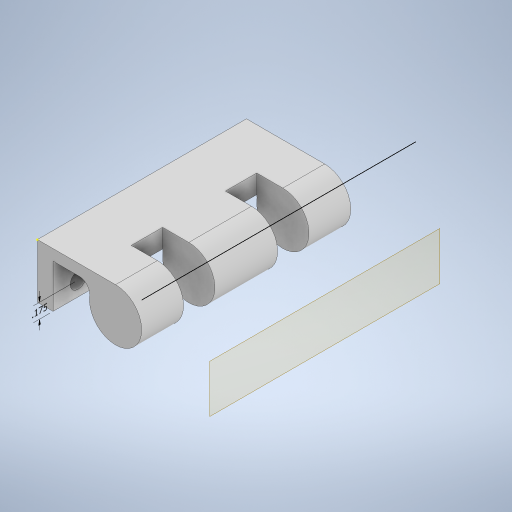
# Autodesk Inventor part: knuckle plate hinge tall
Saved by Autodesk Inventor 2024.2 (Build 282272000, 272)
## iProperties
Created: 2024-08-26
Part Number: knuckle plate hinge tall
Material: Generic
Document SubType Name: Modeling
Designer: Tom
Density: 1 g/cm^3
Appearance: Default
Author: Tom
Autodesk Inventor part; units mm, degrees
ref_plane "YZ Plane" through (0, 0, 0) normal (1, 0, 0) x (0, 1, 0)
ref_plane "XZ Plane" through (0, 0, 0) normal (0, 1, 0) x (-1, 0, 0)
ref_plane "XY Plane" through (0, 0, 0) normal (0, 0, 1) x (1, 0, 0)
sketch "Sketch1" plane through (0, 0, 0) normal (1, 0, 0) x (0, 1, 0)
  line L0 (0, 0) -> (16.51, 0)
  line L1 (16.51, 0) -> (16.51, -63.5)
  line L2 (16.51, -63.5) -> (0, -63.5)
  line L3 (0, -63.5) -> (0, 0)
  circle A0 centre (4.445, -7.62) radius 2.4329
  circle A1 centre (4.445, -15.6185) radius 2.4329
  circle A2 centre (4.445, -23.6169) radius 2.4329
  circle A3 centre (4.445, -31.6154) radius 2.4329
  circle A4 centre (4.445, -39.6138) radius 2.4329
  circle A5 centre (4.445, -47.6123) radius 2.4329
  circle A6 centre (4.445, -55.6108) radius 2.4329
  dimension "d0" = 63.5
  dimension "d1" = 16.51
  dimension "d6" = 7.9985
  dimension "d11" = 7.62
  constraints: 8 end point, 7 centre point, 2 parallel, 1 horizontal, 1 perpendicular, 1 vertical, 12 other
  measures "d0" distance of L0.end L1.end
  measures "d1" distance of L0.start L0.end
  measures "d6" distance of A0.centre A1.centre
  measures "d11" distance from line of L0 A0.centre
extrude "Extrusion1" add sketch "Sketch1" along normal blind 4.7625
sketch "Sketch2" plane through (4.7625, 0, 0) normal (1, 0, 0) x (0, 0, -1)
  line L0 (63.5, 16.51) -> (0, 16.51) projected
  line L1 (63.5, 0) -> (63.5, 16.51) projected
  line L2 (0, 16.51) -> (63.5, 16.51)
  line L3 (63.5, 16.51) -> (63.5, 13.208)
  line L4 (63.5, 13.208) -> (0, 13.208)
  line L5 (0, 13.208) -> (0, 16.51)
  point P0 (0, 0)
  dimension "d14" = 3.302
  constraints: 8 end point, 2 parallel, 1 horizontal, 1 perpendicular, 1 point on line
  measures "d14" distance between parallel lines of L4 L0
extrude "Extrusion2" add sketch "Sketch2" along normal blind 1.016
sketch "Sketch3" plane through (0, 0, 0) normal (0, 0, 1) x (1, 0, 0)
  line L0 (5.7785, 16.51) -> (5.7785, 13.208) projected
  arc A0 (15.8804, 9.6157) -> (23.749, 16.51) centre (23.749, 8.5725) ccw
  line L1 (0, 16.51) -> (0, 0) projected
  line L2 (5.7785, 16.51) -> (23.749, 16.51)
  line L3 (4.7625, 13.208) -> (5.7785, 13.208) projected
  line L4 (5.7785, 13.208) -> (12.7329, 13.208)
  arc A1 (15.8804, 9.6157) -> (12.7329, 13.208) centre (12.7329, 10.033) ccw
  point P0 (17.3057, 13.208)
  point P1 (9.5258, 13.208)
  dimension "d17" = 23.749
  dimension "d18" = 15.875
  dimension "d19" = 3.175
  constraints: 5 point on circle, 4 end point, 3 tangent, 2 centre point, 1 collinear, 1 horizontal, 1 point on line
  measures "d17" distance from line of L1 A0.centre
  measures "d18" diameter of A0
  measures "d19" radius of A1
extrude "Extrusion3" add sketch "Sketch3" against normal blind 63.5
sketch "Sketch4" plane through (0, 16.51, 0) normal (0, 1, 0) x (1, 0, 0)
  line L0 (31.6865, 0) -> (31.6865, 63.5) projected
  line L1 (31.6865, 0) -> (31.6865, 83.2403)
  point P0 (0, 0)
  constraints: 2 end point, 1 point on line, 1 vertical
ref_plane "Work Plane1" through (55.5625, 0, 0) normal (1, 0, 0) x (0, 0, -1)
sketch "Sketch6" plane through (0, 16.51, 0) normal (0, 1, 0) x (1, 0, 0)
  line L0 (31.6865, 0) -> (31.6865, 63.5) projected
  line L1 (15.8115, 50.8) -> (31.6865, 50.8)
  line L2 (31.6865, 50.8) -> (31.6865, 41.275)
  line L3 (31.6865, 41.275) -> (15.8115, 41.275)
  line L4 (15.8115, 41.275) -> (15.8115, 50.8)
  line L5 (31.6865, 63.5) -> (15.8115, 63.5) projected
  line L6 (15.8115, 22.225) -> (31.6865, 22.225)
  line L7 (31.6865, 22.225) -> (31.6865, 12.7)
  line L8 (31.6865, 12.7) -> (15.8115, 12.7)
  line L9 (15.8115, 12.7) -> (15.8115, 22.225)
  line L10 (15.8115, 0) -> (31.6865, 0) projected
  point P0 (0, 0)
  point P1 (15.8804, 63.5)
  point P2 (15.8804, 0)
  dimension "d26" = 9.525
  dimension "d27" = 12.7
  dimension "d28" = 9.525
  dimension "d29" = 12.7
  dimension "d32" = 15.875
  dimension "d33" = 15.875
  constraints: 16 end point, 4 parallel, 2 horizontal, 2 perpendicular, 2 point on line
  measures "d26" distance between parallel lines of L3 L1
  measures "d27" distance between parallel lines of L5 L1
  measures "d28" distance between parallel lines of L8 L6
  measures "d29" distance between parallel lines of L10 L8
  measures "d32" distance between parallel lines of L4 L0
  measures "d33" distance between parallel lines of L9 L0
extrude "Extrusion4" cut sketch "Sketch6" against normal through all
body "Solid1"
